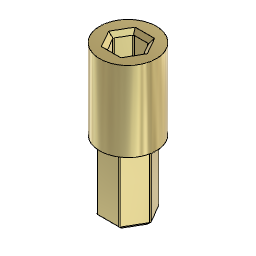
CR-V to Hex Bit Adapter (Autodesk Fusion 360 design; units mm, degrees)
Autodesk Fusion 360 part; units mm, degrees
sketch "Sketch1" plane through (0, 0, 0) normal (0, 0, 1) x (1, 0, 0)
  line L0 (3.8275, 0) -> (1.9137, 3.3147)
  line L1 (1.9137, 3.3147) -> (-1.9137, 3.3147)
  line L2 (-1.9137, 3.3147) -> (-3.8275, 0)
  line L3 (-3.8275, 0) -> (-1.9137, -3.3147)
  line L4 (-1.9137, -3.3147) -> (1.9137, -3.3147)
  line L5 (1.9137, -3.3147) -> (3.8275, 0)
  line L6 (0, 0) -> (0, -3.3147) construction
  dimension "d1" = 6.6294
  constraint coincident L6.start origin
  constraint midpoint L4 L6.end
  constraint vertical L6
  measures "d1" distance of L2 L5
extrude "Extrude1" add sketch "Sketch1" along normal blind 11.43
sketch "Sketch2" plane through (0, 0, 11.43) normal (0, 0, 1) x (-1, 0, 0)
  line L0 (-1.9137, 3.3147) -> (-3.8275, 0)
  line L1 (-3.8275, 0) -> (-1.9137, -3.3147)
  line L2 (-1.9137, -3.3147) -> (1.9137, -3.3147)
  line L3 (1.9137, -3.3147) -> (3.8275, 0)
  line L4 (3.8275, 0) -> (1.9137, 3.3147)
  line L5 (1.9137, 3.3147) -> (-1.9137, 3.3147)
  line L6 (-2.515, 0) -> (-1.2575, -2.1781)
  line L7 (-1.2575, -2.1781) -> (1.2575, -2.1781)
  line L8 (1.2575, -2.1781) -> (2.515, 0)
  line L9 (2.515, 0) -> (1.2575, 2.1781)
  line L10 (1.2575, 2.1781) -> (-1.2575, 2.1781)
  line L11 (-1.2575, 2.1781) -> (-2.515, 0)
  line L12 (0, 2.1781) -> (0, 0) construction
  line L13 (-2.724, 4.7181) -> (-5.4479, 0) construction
  line L14 (-5.4479, 0) -> (-2.724, -4.718) construction
  line L15 (-2.724, -4.718) -> (2.724, -4.718) construction
  line L16 (2.724, -4.718) -> (5.4479, 0) construction
  line L17 (5.4479, 0) -> (2.724, 4.7181) construction
  line L18 (2.724, 4.7181) -> (-2.724, 4.7181) construction
  circle A0 centre (0, 0) radius 4.7181
  dimension "d5" = 4.3561
  dimension "d6" = 2.54
  constraint coincident L12.end A0.centre
  constraint midpoint L10 L12.start
  constraint vertical L12
  constraint tangent L18 A0
  measures "d5" distance of L8 L11
extrude "Extrude2" add sketch "Sketch2" along normal blind 13.335 contours L0 L1 L2 L3 L4 L5 | A0
chamfer "Chamfer1" distance 0.635 angle 45 6 edges at (0, -2.1781, 24.765) (-1.8862, -1.089, 24.765) (-1.8862, 1.089, 24.765) (0, 2.1781, 24.765) (1.8862, 1.089, 24.765) (1.8862, -1.089, 24.765) 1 faces at (1.2758, 0, 0)
fillet "Fillet1" radius 0.2858 12 edges at (-3.8275, 0, 6.0325) (-1.9137, -3.3147, 6.0325) (1.9137, -3.3147, 6.0325) (-1.9137, 3.3147, 6.0325) (1.9137, 3.3147, 6.0325) (3.8275, 0, 6.0325) (2.515, 0, 17.78) (1.2575, -2.1781, 17.78) (-1.2575, -2.1781, 17.78) (-2.515, 0, 17.78) (-1.2575, 2.1781, 17.78) (1.2575, 2.1781, 17.78)
chamfer "Chamfer2" distance 0.381 angle 45 12 edges at (2.8706, 1.6574, 11.43) (1.8916, 3.2764, 11.43) (0, 3.3147, 11.43) (-1.8916, 3.2764, 11.43) (-2.8706, 1.6574, 11.43) (-3.7833, 0, 11.43) (-2.8706, -1.6574, 11.43) (-1.8916, -3.2764, 11.43) (0, -3.3147, 11.43) (1.8916, -3.2764, 11.43) (2.8706, -1.6574, 11.43) (3.7833, 0, 11.43)
chamfer "Chamfer3" distance 0.2223 angle 45 1 faces at (0.3642, 0.726, 11.43)
equation "d1 = 0.248 in + 0.013 in"
equation "d5 = 0.1565 in + ( 0.015 ) * 1 in"
